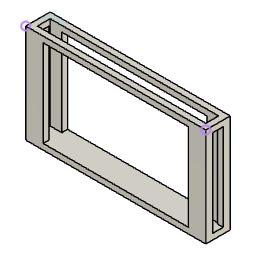
Robot Phone Case (Autodesk Fusion 360 design; units mm, degrees)
Autodesk Fusion 360 part; units mm, degrees
sketch "Sketch1" plane through (0, 0, 0) normal (0, 0, 1) x (1, 0, 0)
  line L0 (0, 0) -> (155, 0)
  line L1 (155, 0) -> (155, 21)
  line L2 (155, 21) -> (0, 21)
  line L3 (0, 21) -> (0, 0)
  dimension "d1" = 155
  dimension "d2" = 21
  constraint horizontal L0
  constraint vertical L1
  constraint horizontal L2
  constraint vertical L3
  constraint coincident L0.start L3.end
  measures "d1" distance of L0.start L0.end
  measures "d2" distance of L0.start L2.end
extrude "Extrude1" add sketch "Sketch1" along normal blind 85
sketch "Sketch2" plane through (0, 0, 85) normal (0, 0, 1) x (-1, 0, 0)
  line L0 (0, -21) -> (0, 0)
  line L1 (-155, 0) -> (-155, -21)
  line L2 (-155, -21) -> (0, -21)
shell "Shell1" thickness 5 removed faces 1 at (51.6667, 7, 85)
sketch "Sketch3" plane through (0, 0, 85) normal (0, 0, 1) x (-1, 0, 0)
sketch "Sketch4" plane through (0, 0, 85) normal (0, 0, 1) x (-1, 0, 0)
sketch "Sketch5" plane through (0, 0, 85) normal (0, 0, 1) x (-1, 0, 0)
sketch "Sketch6" plane through (0, 0, 85) normal (0, 0, 1) x (-1, 0, 0)
sketch "Sketch7" plane through (0, 0, 85) normal (0, 0, 1) x (-1, 0, 0)
sketch "Sketch8" plane through (0, 0, 85) normal (0, 0, 1) x (-1, 0, 0)
sketch "Sketch9" plane through (0, 0, 85) normal (0, 0, 1) x (-1, 0, 0)
sketch "Sketch10" plane through (0, 0, 85) normal (0, 0, 1) x (-1, 0, 0)
  line L0 (-140, 0) -> (-15, 0)
  line L1 (-15, 0) -> (-15, -21)
  line L2 (-15, -21) -> (-140, -21)
  line L3 (-140, -21) -> (-140, 0)
  constraint horizontal L0
  constraint vertical L1
  constraint horizontal L2
  constraint vertical L3
extrude "Extrude2" cut sketch "Sketch10" against normal blind 80
sketch "Sketch11" plane through (0, 0, 85) normal (0, 0, 1) x (-1, 0, 0)
  line L0 (-15, 0) -> (-15, -5)
  line L1 (-15, -5) -> (-5, -5)
  line L2 (-5, -5) -> (-5, -16)
  line L3 (-5, -16) -> (-15, -16)
  line L4 (-15, -16) -> (-15, -21)
  line L5 (-15, -21) -> (0, -21)
  line L6 (0, -21) -> (0, 0)
  line L7 (0, 0) -> (-15, 0)
  line L8 (-6, -13) -> (0, -13)
  line L9 (0, -8) -> (-6, -8)
  line L10 (-6, -13) -> (-155, -13)
  line L11 (-155, -13) -> (-155, -8)
  line L12 (-155, -8) -> (-6, -8)
  line L13 (0, -13) -> (0, -8)
  constraint horizontal L8
  constraint horizontal L9
  constraint coincident L6 L9.start
  constraint horizontal L10
  constraint vertical L11
  constraint horizontal L12
  constraint perpendicular L9 L13
extrude "Extrude3" cut sketch "Sketch11" against normal blind 80 contours L2 L6 L8 L9 L13 | L2 L8 L9 L10 L11 L12
sketch "Sketch12" plane through (0, 0, 85) normal (0, 0, 1) x (-1, 0, 0)
  line L0 (0, -13) -> (-5, -13)
  line L1 (-5, -13) -> (-5, -16)
  line L2 (-5, -16) -> (-15, -16)
  line L3 (-15, -16) -> (-15, -21)
  line L4 (-15, -21) -> (0, -21)
  line L5 (0, -21) -> (0, -13)
sketch "Sketch13" plane through (0, 0, 85) normal (0, 0, 1) x (-1, 0, 0)
  line L0 (0, -15) -> (-185, -15)
  line L1 (-185, -15) -> (-185, -6)
  line L2 (-185, -6) -> (0, -6)
  line L3 (0, -6) -> (0, -15)
  dimension "d10" = 185
  constraint horizontal L0
  constraint vertical L1
  constraint horizontal L2
  constraint vertical L3
  measures "d10" distance of L0.start L0.end
extrude "Extrude4" cut sketch "Sketch13" against normal blind 80
sketch "Sketch14" plane through (15, 0, 0) normal (1, 0, 0) x (0, 1, 0)
  line L0 (5, 5) -> (5, 85)
  line L1 (5, 85) -> (0, 85)
  line L2 (0, 85) -> (0, 5)
  line L3 (0, 5) -> (5, 5)
  line L4 (0, 85) -> (5, 85)
  line L5 (5, 85) -> (5, 80)
  line L6 (5, 80) -> (0, 80)
  line L7 (0, 80) -> (0, 85)
  dimension "d13" = 5
  dimension "d14" = 5
  constraint horizontal L4
  constraint vertical L5
  constraint horizontal L6
  constraint vertical L7
  constraint coincident L1.end L2.start
  measures "d13" distance of L1.end L0.end
  measures "d14" distance of L1.end L6.end
extrude "Extrude5" add sketch "Sketch14" along normal blind 125 contours L0 L1 L2 L4 L5 L6 L7
sketch "Sketch15" plane through (15, 0, 0) normal (1, 0, 0) x (0, 1, 0)
  line L0 (16, 85) -> (16, 5)
  line L1 (16, 5) -> (21, 5)
  line L2 (21, 5) -> (21, 85)
  line L3 (21, 85) -> (16, 85)
  line L4 (21, 85) -> (16, 85)
  line L5 (16, 85) -> (16, 80)
  line L6 (16, 80) -> (21, 80)
  line L7 (21, 80) -> (21, 85)
  dimension "d17" = 5
  constraint horizontal L4
  constraint vertical L5
  constraint horizontal L6
  constraint vertical L7
  constraint coincident L2.end L3.start
  measures "d17" distance of L2.end L6.end
extrude "Extrude6" add sketch "Sketch15" along normal blind 125 contours L0 L2 L3 L4 L5 L6 L7
sketch "Sketch16" plane through (0, 6, 0) normal (0, 1, 0) x (-1, 0, 0)
  line L0 (-5, 85) -> (-5, 5)
  line L1 (-5, 5) -> (0, 5)
  line L2 (0, 5) -> (0, 85)
  line L3 (0, 85) -> (-5, 85)
  line L4 (0, 85) -> (-5, 85)
  line L5 (-5, 85) -> (-5, 80)
  line L6 (-5, 80) -> (0, 80)
  line L7 (0, 80) -> (0, 85)
  dimension "d20" = 5
  constraint horizontal L4
  constraint vertical L5
  constraint horizontal L6
  constraint vertical L7
  constraint coincident L2.end L3.start
  measures "d20" distance of L2.end L6.end
extrude "Extrude7" add sketch "Sketch16" along normal blind 10 contours L0 L2 L3 L4 L5 L6 L7
sketch "Sketch17" plane through (0, 6, 0) normal (0, 1, 0) x (-1, 0, 0)
  line L0 (-150, 5) -> (-150, 85)
  line L1 (-150, 85) -> (-155, 85)
  line L2 (-155, 85) -> (-155, 5)
  line L3 (-155, 5) -> (-150, 5)
  line L4 (-155, 85) -> (-150, 85)
  line L5 (-150, 85) -> (-150, 80)
  line L6 (-150, 80) -> (-155, 80)
  line L7 (-155, 80) -> (-155, 85)
  constraint horizontal L4
  constraint vertical L5
  constraint horizontal L6
  constraint vertical L7
  constraint coincident L0 L5.end
  constraint coincident L1.end L2.start
extrude "Extrude8" add sketch "Sketch17" along normal blind 10 contours L0 L1 L2 L4 L5 L6 L7
